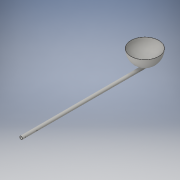
# Autodesk Inventor part: catapultArmWithSaladBowl
Saved by Autodesk Inventor 2016 SP1 (Build 200210100, 210)
## iProperties
Created: 2016-01-16
Part Number: catapultArmWithSaladBowl
Material: Generic
Document SubType Name: Modeling
Designer: steele
Density: 1 g/cm^3
Appearance: Default
Author: steele
Autodesk Inventor part; units mm, degrees
ref_plane "XY Plane" through (0, 0, 0) normal (0, 0, 1) x (1, 0, 0)
sketch "Sketch7" plane through (0, 0, 0) normal (0, 0, 1) x (1, 0, 0)
  circle A0 centre (0, 0) radius 9.525
  circle A1 centre (0, 0) radius 13.97
  dimension "d25" = 27.94
  dimension "d26" = 19.05
  constraints: 2 centre point, 2 coincident
  measures "d25" diameter of A1
  measures "d26" diameter of A0
extrude "Extrusion4" add sketch "Sketch7" along normal blind 1117.6
ref_plane "Work Plane5" through (13.97, 0, 0) normal (1, 0, 0) x (0, 1, 0)
ref_plane "Work Plane6" through (0, 13.97, 0) normal (0, 1, 0) x (-1, 0, 0)
sketch "Sketch9" plane through (0, 13.97, 0) normal (0, 1, 0) x (-1, 0, 0)
  circle A0 centre (0, 25.4) radius 3.302
  line L0 (-13.97, 0) -> (13.97, 0) projected
  point P0 (0, 0)
  dimension "d33" = 25.4
  dimension "d34" = 6.604
  constraints: 1 centre point
  measures "d33" distance from line of A0.centre L0
  measures "d34" diameter of A0
extrude "Extrusion6" cut sketch "Sketch9" against normal through all
sketch "Sketch10" plane through (0, 0, 0) normal (1, 0, 0) x (0, 1, 0)
  arc A0 (13.97, 25.4) -> (137.795, -98.425) centre (137.795, 25.4) ccw
  line L0 (-13.97, 0) -> (13.97, 0) projected
  line L1 (137.795, 25.4) -> (13.97, 25.4) construction
  line L2 (13.97, 0) -> (13.97, 1117.6) construction
  line L3 (137.795, 25.4) -> (137.795, -98.425) construction
  arc A1 (16.51, 25.4) -> (137.795, -95.885) centre (137.795, 25.4) ccw
  line L4 (137.795, -95.885) -> (137.795, -98.425)
  line L5 (16.51, 25.4) -> (13.97, 25.4)
  point P0 (0, 0)
  dimension "d37" = 25.4
  dimension "d38" = 247.65
  dimension "d39" = 123.825
  dimension "d40" = 242.57
  constraints: 8 end point, 4 point on circle, 3 point on line, 2 centre point, 2 collinear, 1 coincident, 1 vertical
  measures "d37" distance from line of L1.start L0
  measures "d38" diameter of A0
  measures "d39" horizontal distance of L0.end L1.start
  measures "d40" diameter of A1
revolve "Revolution4" add sketch "Sketch10" angle 360 about axis through (0, 137.795, 25.4) along (0, -1, 0)
ref_plane "Work Plane7" through (13.97, 0, 0) normal (1, 0, 0) x (0, 1, 0)
sketch "Sketch13" plane through (13.97, 0, 0) normal (1, 0, 0) x (0, 1, 0)
  line L0 (13.97, 1117.6) -> (-13.97, 1117.6) construction
  line L1 (0, 1117.6) -> (0, 0) construction
  line L2 (-13.97, 0) -> (-13.97, 1117.6) construction
  circle A0 centre (0, 1092.2) radius 3.302
  circle A1 centre (0, 990.6) radius 3.175
  dimension "d59" = 25.4
  dimension "d60" = 127
  dimension "d61" = 6.604
  dimension "d62" = 6.35
  constraints: 2 centre point, 2 end point, 2 point on line, 1 midpoint, 1 parallel
  measures "d59" distance of A0.centre L1.start
  measures "d60" distance of A1.centre L1.start
  measures "d61" diameter of A0
  measures "d62" diameter of A1
extrude "Extrusion7" cut sketch "Sketch13" against normal through all
equation "\"d25\" = ballHolderPipeOutsideDiam"
equation "\"d26\" = ballHolderPipeInsideDiam"
equation "\"d27\" = ballHolderLoopHandleLength"
equation "\"d33\" = catapulutArmSaldBoleHoleDistanceFromEnd"
equation "\"d34\" = catapultArmSaladBowlHoleDiam"
equation "\"d35\" = ballHolderLoopHandleLength"
equation "\"d37\" = catapulutArmSaldBoleHoleDistanceFromEnd"
equation "\"d38\" = ballDiam"
equation "\"d39\" = ballRadius"
equation "\"d40\" = -2 * saladHolderThickness + 2 * ballRadius"
equation "\"d59\" = ballHolderAxelDistanceFromEnd"
equation "\"d60\" = holeForAirCylinderDistanceFromEnd"
equation "\"d61\" = ballHolderAxelDiam"
equation "\"d62\" = holeForAirCylinderDiam"
equation "\"d63\" = ballHolderLoopHandleLength"
equation "\"ballHolderLoopDiam\" = 203.2"
equation "\"ballHolderLoopHandleLength\" = 1117.6"
equation "\"xxx\" = 0.5 * ballHolderLoopDiam + ballHolderLoopHandleLength"
equation "\"ballHolderPipeInsideDiam\" = 19.05"
equation "\"ballHolderPipeOutsideDiam\" = 27.94"
equation "\"ballHolderLoopRadius\" = 0.5 * ballHolderLoopDiam"
equation "\"ballHolderAxelDiam\" = 6.604"
equation "\"ballHolderAxelDistanceFromEnd\" = 25.4"
equation "\"catapultArmSaladBowlHoleDiam\" = 6.604"
equation "\"catapulutArmSaldBoleHoleDistanceFromEnd\" = 25.4"
equation "\"ballDiam\" = 247.65"
equation "\"ballRadius\" = 0.5 * ballDiam"
equation "\"saladHolderThickness\" = 2.54"
equation "\"holeForAirCylinderDiam\" = 6.35"
equation "\"holeForAirCylinderDistanceFromEnd\" = 127"
equation "\"d58\" = 0.5 * ballHolderPipeOutsideDiam"
body "Solid3"
